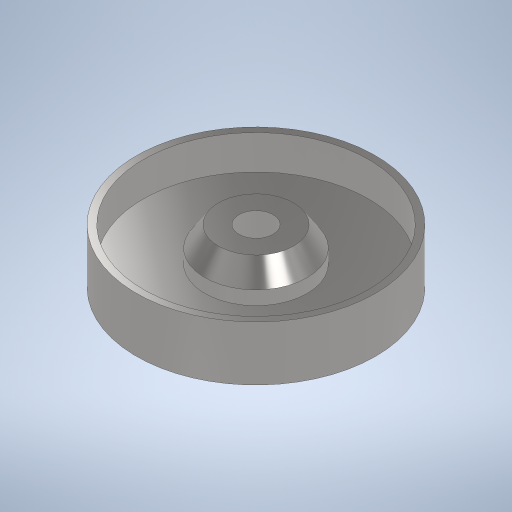
# Autodesk Inventor part: Base
Saved by Autodesk Inventor 2023.2 (Build 272271000, 271)
## iProperties
Created: 2023-03-04
Part Number: Base
Material: Stainless Steel
Document SubType Name: Modeling
Designer: Nathan Cai
Density: 8 g/cm^3
Appearance: Semi-Polished
Author: Nathan Cai
Autodesk Inventor part; units mm, degrees
ref_plane "YZ Plane" through (0, 0, 0) normal (1, 0, 0) x (0, 1, 0)
ref_plane "XZ Plane" through (0, 0, 0) normal (0, 1, 0) x (-1, 0, 0)
ref_plane "XY Plane" through (0, 0, 0) normal (0, 0, 1) x (1, 0, 0)
sketch "Sketch1" plane through (0, 0, 0) normal (0, 0, 1) x (1, 0, 0)
  line L0 (0, 0) -> (17.5, 0)
  line L1 (17.5, 0) -> (17.5, 8)
  line L2 (17.5, 8) -> (0, 8)
  line L3 (0, 8) -> (0, 0)
  line L4 (0, 8) -> (16.5, 8)
  line L5 (16.5, 8) -> (16.5, 3)
  line L6 (16.5, 3) -> (0, 3)
  line L7 (0, 3) -> (0, 8)
  line L8 (0, 3) -> (7.5, 3)
  line L9 (7.5, 3) -> (7.5, 5)
  line L10 (7.5, 5) -> (0, 5)
  line L11 (0, 5) -> (0, 3)
  line L12 (7.5, 5) -> (5.5, 8)
  line L13 (0, 8) -> (2.5, 8)
  line L14 (2.5, 8) -> (2.5, 0)
  line L15 (2.5, 0) -> (0, 0)
  line L16 (0, 0) -> (0, 8)
  point P0 (16.5, 5.5)
  dimension "d0" = 17.5
  dimension "d1" = 8
  dimension "d2" = 1
  dimension "d3" = 3
  dimension "d4" = 7.5
  dimension "d5" = 2
  dimension "d6" = 5.5
  dimension "d7" = 2.5
  constraints: 34 end point, 8 parallel, 4 horizontal, 4 perpendicular, 2 point on line, 1 midpoint
  measures "d0" distance of L2.end L1.end
  measures "d1" distance of L1.end L0.end
  measures "d2" distance from line of L1 point (16.5, 5.5)
  measures "d3" distance between parallel lines of L0 L6
  measures "d4" distance of L10.end L9.end
  measures "d5" distance of L9.end L8.end
  measures "d6" distance from line of L3 L12.end
  measures "d7" distance of L14.end L15.end
revolve "Revolution1" add sketch "Sketch1" angle 360 about axis through (0, 8, 0) along (0, -1, 0) contours L14 L6 L5 L2 L1 L0 | L14 L10 L9 L6 | L14 L2 L12 L10
body "Solid1"
